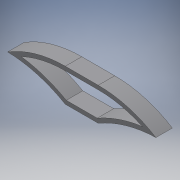
# Autodesk Inventor part: Spring2
Saved by Autodesk Inventor 2016 SP2 (Build 200236200, 236)
## iProperties
Created: 2018-09-27
Part Number: Spring2
Material: Generisch
Document SubType Name: Modeling
Designer: Nils
Density: 1 g/cm^3
Appearance: Vorgabe
Author: Nils
Autodesk Inventor part; units mm, degrees
ref_plane "YZ Plane" through (0, 0, 0) normal (1, 0, 0) x (0, 1, 0)
ref_plane "XZ Plane" through (0, 0, 0) normal (0, 1, 0) x (-1, 0, 0)
ref_plane "XY Plane" through (0, 0, 0) normal (0, 0, 1) x (1, 0, 0)
sketch "Skizze1" plane through (0, 0, 0) normal (0, 1, 0) x (-1, 0, 0)
  line L0 (0, 0) -> (-5.0135, 0)
  line L1 (0, 10) -> (-5, 10)
  arc A0 (-5.0135, 0) -> (-22.5, 5) centre (-23.5683, -31.8139) ccw
  arc A1 (-5, 10) -> (-22.5, 5) centre (-5, -23.125) ccw
  line L2 (0, 8.8) -> (-5, 8.8)
  arc A2 (-5, 8.8) -> (-18.3816, 5.8601) centre (-5, -23.125) ccw
  arc A3 (-4.6919, 1.2) -> (-18.3816, 5.8601) centre (-23.5683, -31.8139) ccw
  line L3 (-4.6919, 1.2) -> (0, 1.2)
  line L4 (0, 0) -> (0, 10) construction
  line L5 (0, 0) -> (5.0135, 0)
  line L6 (0, 10) -> (5, 10)
  arc A4 (22.5, 5) -> (5.0135, 0) centre (23.5683, -31.8139) ccw
  arc A5 (22.5, 5) -> (5, 10) centre (5, -23.125) ccw
  line L7 (0, 8.8) -> (5, 8.8)
  arc A6 (18.3816, 5.8601) -> (5, 8.8) centre (5, -23.125) ccw
  arc A7 (18.3816, 5.8601) -> (4.6919, 1.2) centre (23.5683, -31.8139) ccw
  line L8 (4.6919, 1.2) -> (0, 1.2)
  dimension "d0" = 5
  dimension "d1" = 22.5
  dimension "d2" = 5
  dimension "d3" = 5
  dimension "d4" = 5
  dimension "d6" = 1.2
  dimension "d7" = 10
  constraints: 18 end point, 16 point on circle, 8 centre point, 8 symmetric about line, 2 horizontal, 1 tangent, 7 other
  measures "d0" distance of L1.start L1.end
  measures "d1" horizontal distance of A0.end L0.start
  measures "d2" horizontal distance of L1.end L0.start
  measures "d3" vertical distance of A0.end L0.end
  measures "d4" vertical distance of L1.end A0.end
  measures "d6" radial gap between concentric circles of A0 A3
  measures "d7" distance between parallel lines of L6 L5
extrude "Extrusion1" add sketch "Skizze1" along normal blind 5
